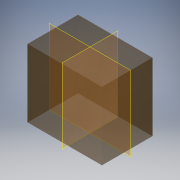
# Autodesk Inventor part: RhinoV19MaxVolume
Saved by Autodesk Inventor 2016 SP1 (Build 200210100, 210)
## iProperties
Created: 2016-02-17
Part Number: RhinoV19MaxVolume
Material: Polycarbonate, Smoke
Document SubType Name: Modeling
Designer: steele
Density: 1.2 g/cm^3
Appearance: Polycarbonate - Smoked
Mass: 31259.1 g
Surface Area: 164470 cm^2
Volume: 26049.3 cm^3
Author: steele
Autodesk Inventor part; units mm, degrees
ref_plane "YZ Plane" through (0, 0, 0) normal (1, 0, 0) x (0, 1, 0)
ref_plane "XZ Plane" through (0, 0, 0) normal (0, 1, 0) x (-1, 0, 0)
ref_plane "XY Plane" through (0, 0, 0) normal (0, 0, 1) x (1, 0, 0)
sketch "Sketch2" plane through (0, 0, 0) normal (0, 1, 0) x (-1, 0, 0)
  line L0 (-749.3, 508) -> (-749.3, -508)
  line L1 (-749.3, -508) -> (749.3, -508)
  line L2 (749.3, -508) -> (749.3, 508)
  line L3 (749.3, 508) -> (-749.3, 508)
  line L4 (-749.3, 508) -> (749.3, -508) construction
  line L5 (-749.3, -508) -> (749.3, 508) construction
  line L6 (-752.475, 511.175) -> (-752.475, -511.175)
  line L7 (-752.475, -511.175) -> (752.475, -511.175)
  line L8 (752.475, -511.175) -> (752.475, 511.175)
  line L9 (752.475, 511.175) -> (-752.475, 511.175)
  line L10 (-752.475, 511.175) -> (752.475, -511.175) construction
  line L11 (-752.475, -511.175) -> (752.475, 511.175) construction
  point P0 (0, 0)
  dimension "d4" = 1016
  dimension "d5" = 1498.6
  dimension "d6" = 3.175
  dimension "d7" = 3.175
  constraints: 24 end point, 4 midpoint, 4 parallel, 2 perpendicular, 2 vertical
  measures "d4" distance of L0.start L0.end
  measures "d5" distance of L2.end L0.start
  measures "d6" distance between parallel lines of L0 L6
  measures "d7" distance between parallel lines of L3 L9
extrude "Extrusion1" add sketch "Sketch2" along normal blind 1371.6
equation "\"d4\" = maxMatchWidth"
equation "\"d5\" = maxMatchLength"
equation "\"d6\" = modelThickness"
equation "\"d7\" = modelThickness"
equation "\"d8\" = maxMatchHeight"
equation "\"robotLength\" = 736.6"
equation "\"robotWidth\" = 254"
equation "\"robotPerimeter\" = 2 * robotLength + 2 * robotWidth"
equation "\"maxMatchLength\" = robotLength + 2 * matchExtension"
equation "\"matchExtension\" = 381"
equation "\"maxMatchWidth\" = robotWidth + 2 * matchExtension"
equation "\"modelThickness\" = 3.175"
equation "\"maxMatchHeight\" = 1371.6"
body "Solid1"
